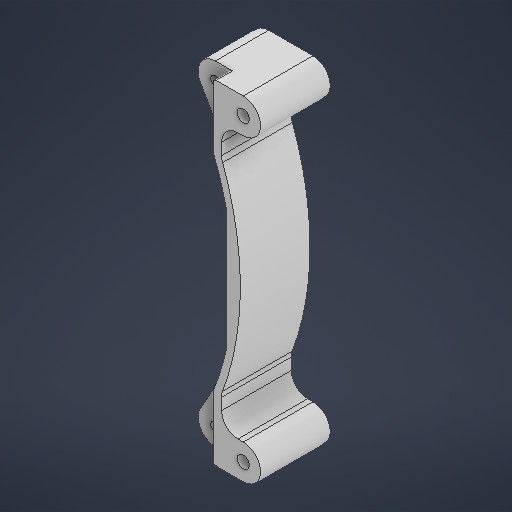
# Autodesk Inventor part: fan_connector_02
Saved by Autodesk Inventor 2026.2 (Build 302298010, 298A)
## iProperties
Created: 2026-05-14
Part Number: fan_connector_02
Material: 一般
Document SubType Name: Modeling
Designer: nyxeon
Density: 1 g/cm^3
Appearance: 既定
Author: nyxeon
Autodesk Inventor part; units mm, degrees
ref_plane "YZ Plane" through (0, 0, 0) normal (1, 0, 0) x (0, 1, 0)
ref_plane "XZ Plane" through (0, 0, 0) normal (0, 1, 0) x (-1, 0, 0)
ref_plane "XY Plane" through (0, 0, 0) normal (0, 0, 1) x (1, 0, 0)
sketch "スケッチ1" plane through (0, 0, 0) normal (0, 0, 1) x (1, 0, 0)
  line L0 (215.8192, 50.162) -> (210.8692, 50.162) construction
  line L1 (210.8692, 59.3371) -> (210.8692, 50.162) construction
  arc A0 (210.8692, 59.3371) -> (210.3611, 60.6691) centre (208.8692, 59.3371) ccw construction
  line L2 (208.3692, 62.9) -> (210.3611, 60.6691) construction
  line L3 (208.3692, 63.9) -> (208.3692, 62.9) construction
  arc A1 (206.8692, 65.4) -> (208.3692, 63.9) centre (208.3692, 65.4) ccw construction
  line L4 (206.8692, 65.4) -> (206.8692, 85.3) construction
  arc A2 (206.8692, 85.3) -> (200.8692, 91.3) centre (200.8692, 85.3) ccw construction
  line L5 (200.8692, 91.3) -> (180.9692, 91.3) construction
  arc A3 (179.4692, 92.8) -> (180.9692, 91.3) centre (180.9692, 92.8) ccw construction
  line L6 (179.4692, 92.8) -> (178.4692, 92.8) construction
  line L7 (178.4692, 92.8) -> (176.2383, 94.7919) construction
  arc A4 (176.2383, 94.7919) -> (174.9063, 95.3) centre (174.9063, 93.3) ccw construction
  line L8 (174.9063, 95.3) -> (153.3073, 95.3) construction
  arc A5 (153.3073, 95.3) -> (136.9278, 100.25) centre (115.5692, 0) ccw construction
  line L9 (94.2107, 100.25) -> (136.9278, 100.25) construction
  arc A6 (94.2107, 100.25) -> (77.8312, 95.3) centre (115.5692, 0) ccw construction
  line L10 (56.2322, 95.3) -> (77.8312, 95.3) construction
  arc A7 (56.2322, 95.3) -> (54.9001, 94.7919) centre (56.2322, 93.3) ccw construction
  line L11 (52.6692, 92.8) -> (54.9001, 94.7919) construction
  line L12 (51.6692, 92.8) -> (52.6692, 92.8) construction
  arc A8 (50.1692, 91.3) -> (51.6692, 92.8) centre (50.1692, 92.8) ccw construction
  line L13 (30.2692, 91.3) -> (50.1692, 91.3) construction
  arc A9 (30.2692, 91.3) -> (24.2692, 85.3) centre (30.2692, 85.3) ccw construction
  line L14 (24.2692, 65.4) -> (24.2692, 85.3) construction
  arc A10 (22.7692, 63.9) -> (24.2692, 65.4) centre (22.7692, 65.4) ccw construction
  line L15 (22.7692, 63.9) -> (22.7692, 62.9) construction
  line L16 (22.7692, 62.9) -> (20.7774, 60.6691) construction
  arc A11 (20.7774, 60.6691) -> (20.2692, 59.3371) centre (22.2692, 59.3371) ccw construction
  line L17 (20.2692, 59.3371) -> (20.2692, 37.738) construction
  arc A12 (20.2692, 37.738) -> (15.3192, 21.3585) centre (115.5692, 0) ccw construction
  line L18 (15.3192, -21.3585) -> (15.3192, 21.3585) construction
  arc A13 (15.3192, -21.3585) -> (20.2692, -37.738) centre (115.5692, 0) ccw construction
  line L19 (20.2692, -59.3371) -> (20.2692, -37.738) construction
  arc A14 (20.2692, -59.3371) -> (20.7774, -60.6691) centre (22.2692, -59.3371) ccw construction
  line L20 (22.7692, -62.9) -> (20.7774, -60.6691) construction
  line L21 (22.7692, -63.9) -> (22.7692, -62.9) construction
  arc A15 (24.2692, -65.4) -> (22.7692, -63.9) centre (22.7692, -65.4) ccw construction
  line L22 (24.2692, -65.4) -> (24.2692, -85.3) construction
  arc A16 (24.2692, -85.3) -> (30.2692, -91.3) centre (30.2692, -85.3) ccw construction
  line L23 (30.2692, -91.3) -> (50.1692, -91.3) construction
  arc A17 (51.6692, -92.8) -> (50.1692, -91.3) centre (50.1692, -92.8) ccw construction
  line L24 (51.6692, -92.8) -> (52.6692, -92.8) construction
  line L25 (52.6692, -92.8) -> (54.9001, -94.7919) construction
  arc A18 (54.9001, -94.7919) -> (56.2322, -95.3) centre (56.2322, -93.3) ccw construction
  line L26 (56.2322, -95.3) -> (77.8312, -95.3) construction
  arc A19 (77.8312, -95.3) -> (94.2107, -100.25) centre (115.5692, 0) ccw construction
  line L27 (94.2107, -100.25) -> (136.9278, -100.25) construction
  arc A20 (136.9278, -100.25) -> (153.3073, -95.3) centre (115.5692, 0) ccw construction
  line L28 (174.9063, -95.3) -> (153.3073, -95.3) construction
  arc A21 (174.9063, -95.3) -> (176.2383, -94.7919) centre (174.9063, -93.3) ccw construction
  line L29 (178.4692, -92.8) -> (176.2383, -94.7919) construction
  line L30 (179.4692, -92.8) -> (178.4692, -92.8) construction
  arc A22 (180.9692, -91.3) -> (179.4692, -92.8) centre (180.9692, -92.8) ccw construction
  line L31 (200.8692, -91.3) -> (180.9692, -91.3) construction
  arc A23 (200.8692, -91.3) -> (206.8692, -85.3) centre (200.8692, -85.3) ccw construction
  line L32 (206.8692, -65.4) -> (206.8692, -85.3) construction
  arc A24 (208.3692, -63.9) -> (206.8692, -65.4) centre (208.3692, -65.4) ccw construction
  line L33 (208.3692, -63.9) -> (208.3692, -62.9) construction
  line L34 (208.3692, -62.9) -> (210.3611, -60.6691) construction
  arc A25 (210.3611, -60.6691) -> (210.8692, -59.3371) centre (208.8692, -59.3371) ccw construction
  line L35 (210.8692, -59.3371) -> (210.8692, -37.738) construction
  arc A26 (210.8692, -37.738) -> (215.8192, -21.3585) centre (115.5692, 0) ccw construction
  line L36 (215.8192, -21.3585) -> (215.8192, 50.162) construction
  circle A27 centre (30.5692, 85) radius 2.2 construction
  circle A28 centre (38.3192, 77.25) radius 2.2 construction
  circle A29 centre (192.8192, -77.25) radius 2.2 construction
  circle A30 centre (200.5692, -85) radius 2.2 construction
  circle A31 centre (170.5692, -90) radius 2.2 construction
  circle A32 centre (200.5817, -67.0124) radius 1.35 construction
  circle A33 centre (205.5692, -55) radius 2.2 construction
  circle A34 centre (182.5817, 85.0124) radius 1.35 construction
  circle A35 centre (192.8192, 77.25) radius 2.2 construction
  circle A36 centre (200.5692, 85) radius 2.2 construction
  circle A37 centre (170.5692, 90) radius 2.2 construction
  circle A38 centre (200.5817, 67.0124) radius 1.35 construction
  circle A39 centre (205.5692, 55) radius 2.2 construction
  circle A40 centre (182.5817, -85.0124) radius 1.35 construction
  circle A41 centre (25.5692, -55) radius 2.2 construction
  circle A42 centre (30.5568, -67.0124) radius 1.35 construction
  circle A43 centre (60.5692, -90) radius 2.2 construction
  circle A44 centre (30.5692, -85) radius 2.2 construction
  circle A45 centre (60.5692, 90) radius 2.2 construction
  circle A46 centre (30.5568, 67.0124) radius 1.35 construction
  circle A47 centre (25.5692, 55) radius 2.2 construction
  circle A48 centre (48.5568, -85.0124) radius 1.35 construction
  circle A49 centre (48.5568, 85.0124) radius 1.35 construction
  circle A50 centre (38.3192, -77.25) radius 2.2 construction
  arc A51 (49.757, -72.8834) -> (93.3332, -95.6494) centre (115.5692, 0) ccw construction
  line L37 (49.757, -72.8834) -> (41.388, -81.2523) construction
  arc A52 (40.2566, -80.121) -> (41.388, -81.2523) centre (40.8223, -80.6866) ccw construction
  line L38 (48.5772, -71.8004) -> (40.2566, -80.121) construction
  arc A53 (43.7688, -66.9921) -> (48.5772, -71.8004) centre (115.5692, 0) ccw construction
  line L39 (43.7688, -66.9921) -> (35.4483, -75.3126) construction
  arc A54 (34.3169, -74.1813) -> (35.4483, -75.3126) centre (34.8826, -74.747) ccw construction
  line L40 (42.6859, -65.8123) -> (34.3169, -74.1813) construction
  arc A55 (19.9199, -22.236) -> (42.6859, -65.8123) centre (115.5692, 0) ccw construction
  line L41 (18.6687, -21) -> (19.9199, -22.236) construction
  arc A56 (18.6687, 21) -> (18.6687, -21) centre (115.5692, 0) ccw construction
  line L42 (18.6687, 21) -> (19.9199, 22.236) construction
  arc A57 (42.6859, 65.8123) -> (19.9199, 22.236) centre (115.5692, 0) ccw construction
  line L43 (42.6859, 65.8123) -> (34.3169, 74.1813) construction
  arc A58 (35.4483, 75.3126) -> (34.3169, 74.1813) centre (34.8826, 74.747) ccw construction
  line L44 (43.7688, 66.9921) -> (35.4483, 75.3126) construction
  arc A59 (48.5772, 71.8004) -> (43.7688, 66.9921) centre (115.5692, 0) ccw construction
  line L45 (48.5772, 71.8004) -> (40.2566, 80.121) construction
  arc A60 (41.388, 81.2523) -> (40.2566, 80.121) centre (40.8223, 80.6866) ccw construction
  line L46 (49.757, 72.8834) -> (41.388, 81.2523) construction
  arc A61 (93.3332, 95.6494) -> (49.757, 72.8834) centre (115.5692, 0) ccw construction
  line L47 (94.5692, 96.9006) -> (93.3332, 95.6494) construction
  arc A62 (136.5692, 96.9006) -> (94.5692, 96.9006) centre (115.5692, 0) ccw construction
  line L48 (136.5692, 96.9006) -> (137.8053, 95.6494) construction
  arc A63 (181.3815, 72.8834) -> (137.8053, 95.6494) centre (115.5692, 0) ccw construction
  line L49 (181.3815, 72.8834) -> (189.7505, 81.2523) construction
  arc A64 (190.8819, 80.121) -> (189.7505, 81.2523) centre (190.3162, 80.6866) ccw construction
  line L50 (182.5613, 71.8004) -> (190.8819, 80.121) construction
  arc A65 (187.3697, 66.9921) -> (182.5613, 71.8004) centre (115.5692, 0) ccw construction
  line L51 (187.3697, 66.9921) -> (195.6902, 75.3126) construction
  arc A66 (196.8216, 74.1813) -> (195.6902, 75.3126) centre (196.2559, 74.747) ccw construction
  line L52 (188.4526, 65.8123) -> (196.8216, 74.1813) construction
  arc A67 (211.2186, 22.236) -> (188.4526, 65.8123) centre (115.5692, 0) ccw construction
  line L53 (212.4698, 21) -> (211.2186, 22.236) construction
  arc A68 (212.4698, -21) -> (212.4698, 21) centre (115.5692, 0) ccw construction
  line L54 (212.4698, -21) -> (211.2186, -22.236) construction
  arc A69 (188.4526, -65.8123) -> (211.2186, -22.236) centre (115.5692, 0) ccw construction
  line L55 (188.4526, -65.8123) -> (196.8216, -74.1813) construction
  arc A70 (195.6902, -75.3126) -> (196.8216, -74.1813) centre (196.2559, -74.747) ccw construction
  line L56 (187.3697, -66.9921) -> (195.6902, -75.3126) construction
  arc A71 (182.5613, -71.8004) -> (187.3697, -66.9921) centre (115.5692, 0) ccw construction
  line L57 (182.5613, -71.8004) -> (190.8819, -80.121) construction
  arc A72 (189.7505, -81.2523) -> (190.8819, -80.121) centre (190.3162, -80.6866) ccw construction
  line L58 (181.3815, -72.8834) -> (189.7505, -81.2523) construction
  arc A73 (137.8053, -95.6494) -> (181.3815, -72.8834) centre (115.5692, 0) ccw construction
  line L59 (136.5692, -96.9006) -> (137.8053, -95.6494) construction
  arc A74 (94.5692, -96.9006) -> (136.5692, -96.9006) centre (115.5692, 0) ccw construction
  line L60 (94.5692, -96.9006) -> (93.3332, -95.6494) construction
  line L61 (12.0692, 50.162) -> (7.1192, 50.162) construction
  line L62 (7.1192, 59.3371) -> (7.1192, 50.162) construction
  arc A75 (7.1192, 59.3371) -> (6.6111, 60.6691) centre (5.1192, 59.3371) ccw construction
  line L63 (4.6192, 62.9) -> (6.6111, 60.6691) construction
  line L64 (4.6192, 63.9) -> (4.6192, 62.9) construction
  arc A76 (3.1192, 65.4) -> (4.6192, 63.9) centre (4.6192, 65.4) ccw construction
  line L65 (3.1192, 65.4) -> (3.1192, 85.3) construction
  arc A77 (3.1192, 85.3) -> (-2.8808, 91.3) centre (-2.8808, 85.3) ccw construction
  line L66 (-2.8808, 91.3) -> (-22.7808, 91.3) construction
  arc A78 (-24.2808, 92.8) -> (-22.7808, 91.3) centre (-22.7808, 92.8) ccw construction
  line L67 (-24.2808, 92.8) -> (-25.2808, 92.8) construction
  line L68 (-25.2808, 92.8) -> (-27.5117, 94.7919) construction
  arc A79 (-27.5117, 94.7919) -> (-28.8437, 95.3) centre (-28.8437, 93.3) ccw construction
  line L69 (-28.8437, 95.3) -> (-50.4427, 95.3) construction
  arc A80 (-50.4427, 95.3) -> (-66.8222, 100.25) centre (-88.1808, 0) ccw construction
  line L70 (-109.5393, 100.25) -> (-66.8222, 100.25) construction
  arc A81 (-109.5393, 100.25) -> (-125.9188, 95.3) centre (-88.1808, 0) ccw construction
  line L71 (-147.5178, 95.3) -> (-125.9188, 95.3) construction
  arc A82 (-147.5178, 95.3) -> (-148.8499, 94.7919) centre (-147.5178, 93.3) ccw construction
  line L72 (-151.0808, 92.8) -> (-148.8499, 94.7919) construction
  line L73 (-152.0808, 92.8) -> (-151.0808, 92.8) construction
  arc A83 (-153.5808, 91.3) -> (-152.0808, 92.8) centre (-153.5808, 92.8) ccw construction
  line L74 (-173.4808, 91.3) -> (-153.5808, 91.3) construction
  arc A84 (-173.4808, 91.3) -> (-179.4808, 85.3) centre (-173.4808, 85.3) ccw construction
  line L75 (-179.4808, 65.4) -> (-179.4808, 85.3) construction
  arc A85 (-180.9808, 63.9) -> (-179.4808, 65.4) centre (-180.9808, 65.4) ccw construction
  line L76 (-180.9808, 63.9) -> (-180.9808, 62.9) construction
  line L77 (-180.9808, 62.9) -> (-182.9726, 60.6691) construction
  arc A86 (-182.9726, 60.6691) -> (-183.4808, 59.3371) centre (-181.4808, 59.3371) ccw construction
  line L78 (-183.4808, 59.3371) -> (-183.4808, 37.738) construction
  arc A87 (-183.4808, 37.738) -> (-188.4308, 21.3585) centre (-88.1808, 0) ccw construction
  line L79 (-188.4308, -21.3585) -> (-188.4308, 21.3585) construction
  arc A88 (-188.4308, -21.3585) -> (-183.4808, -37.738) centre (-88.1808, 0) ccw construction
  line L80 (-183.4808, -59.3371) -> (-183.4808, -37.738) construction
  arc A89 (-183.4808, -59.3371) -> (-182.9726, -60.6691) centre (-181.4808, -59.3371) ccw construction
  line L81 (-180.9808, -62.9) -> (-182.9726, -60.6691) construction
  line L82 (-180.9808, -63.9) -> (-180.9808, -62.9) construction
  arc A90 (-179.4808, -65.4) -> (-180.9808, -63.9) centre (-180.9808, -65.4) ccw construction
  line L83 (-179.4808, -65.4) -> (-179.4808, -85.3) construction
  arc A91 (-179.4808, -85.3) -> (-173.4808, -91.3) centre (-173.4808, -85.3) ccw construction
  line L84 (-173.4808, -91.3) -> (-153.5808, -91.3) construction
  arc A92 (-152.0808, -92.8) -> (-153.5808, -91.3) centre (-153.5808, -92.8) ccw construction
  line L85 (-152.0808, -92.8) -> (-151.0808, -92.8) construction
  line L86 (-151.0808, -92.8) -> (-148.8499, -94.7919) construction
  arc A93 (-148.8499, -94.7919) -> (-147.5178, -95.3) centre (-147.5178, -93.3) ccw construction
  line L87 (-147.5178, -95.3) -> (-125.9188, -95.3) construction
  arc A94 (-125.9188, -95.3) -> (-109.5393, -100.25) centre (-88.1808, 0) ccw construction
  line L88 (-109.5393, -100.25) -> (-66.8222, -100.25) construction
  arc A95 (-66.8222, -100.25) -> (-50.4427, -95.3) centre (-88.1808, 0) ccw construction
  line L89 (-28.8437, -95.3) -> (-50.4427, -95.3) construction
  arc A96 (-28.8437, -95.3) -> (-27.5117, -94.7919) centre (-28.8437, -93.3) ccw construction
  line L90 (-25.2808, -92.8) -> (-27.5117, -94.7919) construction
  line L91 (-24.2808, -92.8) -> (-25.2808, -92.8) construction
  arc A97 (-22.7808, -91.3) -> (-24.2808, -92.8) centre (-22.7808, -92.8) ccw construction
  line L92 (-2.8808, -91.3) -> (-22.7808, -91.3) construction
  arc A98 (-2.8808, -91.3) -> (3.1192, -85.3) centre (-2.8808, -85.3) ccw construction
  line L93 (3.1192, -65.4) -> (3.1192, -85.3) construction
  arc A99 (4.6192, -63.9) -> (3.1192, -65.4) centre (4.6192, -65.4) ccw construction
  line L94 (4.6192, -63.9) -> (4.6192, -62.9) construction
  line L95 (4.6192, -62.9) -> (6.6111, -60.6691) construction
  arc A100 (6.6111, -60.6691) -> (7.1192, -59.3371) centre (5.1192, -59.3371) ccw construction
  line L96 (7.1192, -59.3371) -> (7.1192, -37.738) construction
  arc A101 (7.1192, -37.738) -> (12.0692, -21.3585) centre (-88.1808, 0) ccw construction
  line L97 (12.0692, -21.3585) -> (12.0692, 50.162) construction
  circle A102 centre (-173.1808, 85) radius 2.2 construction
  circle A103 centre (-165.4308, 77.25) radius 2.2 construction
  circle A104 centre (-10.9308, -77.25) radius 2.2 construction
  circle A105 centre (-3.1808, -85) radius 2.2 construction
  circle A106 centre (-33.1808, -90) radius 2.2 construction
  circle A107 centre (-3.1683, -67.0124) radius 1.35 construction
  circle A108 centre (1.8192, -55) radius 2.2 construction
  circle A109 centre (-21.1683, 85.0124) radius 1.35 construction
  circle A110 centre (-10.9308, 77.25) radius 2.2 construction
  circle A111 centre (-3.1808, 85) radius 2.2 construction
  circle A112 centre (-33.1808, 90) radius 2.2 construction
  circle A113 centre (-3.1683, 67.0124) radius 1.35 construction
  circle A114 centre (1.8192, 55) radius 2.2 construction
  circle A115 centre (-21.1683, -85.0124) radius 1.35 construction
  circle A116 centre (-178.1808, -55) radius 2.2 construction
  circle A117 centre (-173.1932, -67.0124) radius 1.35 construction
  circle A118 centre (-143.1808, -90) radius 2.2 construction
  circle A119 centre (-173.1808, -85) radius 2.2 construction
  circle A120 centre (-143.1808, 90) radius 2.2 construction
  circle A121 centre (-173.1932, 67.0124) radius 1.35 construction
  circle A122 centre (-178.1808, 55) radius 2.2 construction
  circle A123 centre (-155.1932, -85.0124) radius 1.35 construction
  circle A124 centre (-155.1932, 85.0124) radius 1.35 construction
  circle A125 centre (-165.4308, -77.25) radius 2.2 construction
  arc A126 (-153.993, -72.8834) -> (-110.4168, -95.6494) centre (-88.1808, 0) ccw construction
  line L98 (-153.993, -72.8834) -> (-162.362, -81.2523) construction
  arc A127 (-163.4934, -80.121) -> (-162.362, -81.2523) centre (-162.9277, -80.6866) ccw construction
  line L99 (-155.1728, -71.8004) -> (-163.4934, -80.121) construction
  arc A128 (-159.9812, -66.9921) -> (-155.1728, -71.8004) centre (-88.1808, 0) ccw construction
  line L100 (-159.9812, -66.9921) -> (-168.3017, -75.3126) construction
  arc A129 (-169.4331, -74.1813) -> (-168.3017, -75.3126) centre (-168.8674, -74.747) ccw construction
  line L101 (-161.0641, -65.8123) -> (-169.4331, -74.1813) construction
  arc A130 (-183.8301, -22.236) -> (-161.0641, -65.8123) centre (-88.1808, 0) ccw construction
  line L102 (-185.0813, -21) -> (-183.8301, -22.236) construction
  arc A131 (-185.0813, 21) -> (-185.0813, -21) centre (-88.1808, 0) ccw construction
  line L103 (-185.0813, 21) -> (-183.8301, 22.236) construction
  arc A132 (-161.0641, 65.8123) -> (-183.8301, 22.236) centre (-88.1808, 0) ccw construction
  line L104 (-161.0641, 65.8123) -> (-169.4331, 74.1813) construction
  arc A133 (-168.3017, 75.3126) -> (-169.4331, 74.1813) centre (-168.8674, 74.747) ccw construction
  line L105 (-159.9812, 66.9921) -> (-168.3017, 75.3126) construction
  arc A134 (-155.1728, 71.8004) -> (-159.9812, 66.9921) centre (-88.1808, 0) ccw construction
  line L106 (-155.1728, 71.8004) -> (-163.4934, 80.121) construction
  arc A135 (-162.362, 81.2523) -> (-163.4934, 80.121) centre (-162.9277, 80.6866) ccw construction
  line L107 (-153.993, 72.8834) -> (-162.362, 81.2523) construction
  arc A136 (-110.4168, 95.6494) -> (-153.993, 72.8834) centre (-88.1808, 0) ccw construction
  line L108 (-109.1808, 96.9006) -> (-110.4168, 95.6494) construction
  arc A137 (-67.1808, 96.9006) -> (-109.1808, 96.9006) centre (-88.1808, 0) ccw construction
  line L109 (-67.1808, 96.9006) -> (-65.9447, 95.6494) construction
  arc A138 (-22.3685, 72.8834) -> (-65.9447, 95.6494) centre (-88.1808, 0) ccw construction
  line L110 (-22.3685, 72.8834) -> (-13.9995, 81.2523) construction
  arc A139 (-12.8681, 80.121) -> (-13.9995, 81.2523) centre (-13.4338, 80.6866) ccw construction
  line L111 (-21.1887, 71.8004) -> (-12.8681, 80.121) construction
  arc A140 (-16.3803, 66.9921) -> (-21.1887, 71.8004) centre (-88.1808, 0) ccw construction
  line L112 (-16.3803, 66.9921) -> (-8.0598, 75.3126) construction
  arc A141 (-6.9284, 74.1813) -> (-8.0598, 75.3126) centre (-7.4941, 74.747) ccw construction
  line L113 (-15.2974, 65.8123) -> (-6.9284, 74.1813) construction
  arc A142 (7.4686, 22.236) -> (-15.2974, 65.8123) centre (-88.1808, 0) ccw construction
  line L114 (8.7198, 21) -> (7.4686, 22.236) construction
  arc A143 (8.7198, -21) -> (8.7198, 21) centre (-88.1808, 0) ccw construction
  line L115 (8.7198, -21) -> (7.4686, -22.236) construction
  arc A144 (-15.2974, -65.8123) -> (7.4686, -22.236) centre (-88.1808, 0) ccw construction
  line L116 (-15.2974, -65.8123) -> (-6.9284, -74.1813) construction
  arc A145 (-8.0598, -75.3126) -> (-6.9284, -74.1813) centre (-7.4941, -74.747) ccw construction
  line L117 (-16.3803, -66.9921) -> (-8.0598, -75.3126) construction
  arc A146 (-21.1887, -71.8004) -> (-16.3803, -66.9921) centre (-88.1808, 0) ccw construction
  line L118 (-21.1887, -71.8004) -> (-12.8681, -80.121) construction
  arc A147 (-13.9995, -81.2523) -> (-12.8681, -80.121) centre (-13.4338, -80.6866) ccw construction
  line L119 (-22.3685, -72.8834) -> (-13.9995, -81.2523) construction
  arc A148 (-65.9447, -95.6494) -> (-22.3685, -72.8834) centre (-88.1808, 0) ccw construction
  line L120 (-67.1808, -96.9006) -> (-65.9447, -95.6494) construction
  arc A149 (-109.1808, -96.9006) -> (-67.1808, -96.9006) centre (-88.1808, 0) ccw construction
  line L121 (-109.1808, -96.9006) -> (-110.4168, -95.6494) construction
  arc A150 (-14.8018, -66.3079) -> (8.3934, -21.3225) centre (-88.1808, 0) ccw construction
  arc A151 (18.9951, -21.3225) -> (42.1903, -66.3079) centre (115.5692, 0) ccw construction
  line L122 (-88.1808, 0) -> (115.5692, 0) construction
  circle A152 centre (1.8192, -55) radius 6.3251 construction
  circle A153 centre (25.5692, -55) radius 6.3251 construction
  arc A154 (18.6687, -21) -> (94.5692, -96.9006) centre (115.5692, 0) ccw construction
  circle A155 centre (1.8192, 55) radius 6.3251 construction
  circle A156 centre (25.5692, 55) radius 6.3251 construction
  line L123 (25.5692, -55) -> (115.5692, 0) construction
  arc A157 (30.9663, 51.7018) -> (30.9663, -51.7018) centre (115.5692, 0) ccw
  arc A158 (-3.5779, -51.7018) -> (-3.5779, 51.7018) centre (-88.1808, 0) ccw
  arc A159 (25.5692, -61.3251) -> (30.9663, -51.7018) centre (25.5692, -55) ccw
  arc A160 (-3.5779, -51.7018) -> (1.8192, -61.3251) centre (1.8192, -55) ccw
  arc A161 (1.8192, 61.3251) -> (-3.5779, 51.7018) centre (1.8192, 55) ccw
  arc A162 (30.9663, 51.7018) -> (25.5692, 61.3251) centre (25.5692, 55) ccw
  line L124 (1.8192, -61.3251) -> (25.5692, -61.3251)
  line L125 (1.8192, 61.3251) -> (25.5692, 61.3251)
  circle A163 centre (1.8192, -55) radius 1.7
  circle A164 centre (25.5692, -55) radius 1.7
  circle A165 centre (25.5692, 55) radius 1.7
  circle A166 centre (1.8192, 55) radius 1.7
  line L126 (16.4192, 61.3251) -> (16.4192, -61.3251)
  point P0 (0, 0)
  dimension "d0" = 12.6502
  dimension "d1" = 3.4
  constraints: 26 point on circle, 16 centre point, 15 coincident, 10 end point, 5 equal radius, 3 concentric, 3 point on line, 3 tangent, 2 horizontal, 1 horizontal alignment, 1 parallel, 1 vertical, 1 vertical alignment, 11 other
  measures "d0" diameter of A152
  measures "d1" diameter of A163
extrude "押し出し1" add sketch "スケッチ1" along normal blind 15.8 and the other way blind 3.8 contours L126 L124 A160 A158 A161 L125
sketch "スケッチ2" plane through (0, 0, 15.8) normal (0, 0, 1) x (1, 0, 0)
  arc A0 (-270.5722, -100.25) -> (-254.1927, -95.3) centre (-291.9308, 0) ccw construction
  circle A1 centre (18.0692, -55) radius 2.25
  line L0 (7.1192, -59.3371) -> (7.1192, -37.738) projected
  arc A2 (7.1192, -37.738) -> (12.0692, -21.3585) centre (-88.1808, 0) ccw projected
  line L1 (12.0692, -21.3585) -> (12.0692, 21.3585) projected
  arc A3 (12.0692, 21.3585) -> (7.1192, 37.738) centre (-88.1808, 0) ccw projected
  line L2 (7.1192, 59.3371) -> (7.1192, 37.738) projected
  arc A4 (7.1192, 59.3371) -> (6.6111, 60.6691) centre (5.1192, 59.3371) ccw projected
  line L3 (4.6192, 62.9) -> (6.6111, 60.6691) projected
  arc A5 (6.6111, -60.6691) -> (7.1192, -59.3371) centre (5.1192, -59.3371) ccw projected
  line L4 (4.6192, -62.9) -> (6.6111, -60.6691) projected
  line L5 (16.4192, -61.3251) -> (16.4192, 61.3251) projected
  line L6 (16.4192, 61.3251) -> (1.8192, 61.3251) projected
  line L7 (1.8192, -61.3251) -> (16.4192, -61.3251) projected
  circle A6 centre (1.8192, -55) radius 1.7 construction
  circle A7 centre (1.8192, 55) radius 1.7 construction
  arc A8 (-3.5779, -51.7018) -> (1.8192, -61.3251) centre (1.8192, -55) ccw construction
  circle A9 centre (18.0692, -55) radius 6.3251 construction
  line L8 (16.4192, -61.3251) -> (18.0692, -61.3251)
  line L9 (7.1192, -59.3371) -> (7.1192, -61.3251)
  circle A10 centre (18.0692, 55) radius 2.25
  circle A11 centre (18.0692, 55) radius 6.3251 construction
  line L10 (7.1192, 59.3371) -> (7.1192, 61.3251)
  line L11 (16.4192, 61.3251) -> (18.0692, 61.3251)
  line L12 (24.3944, 55) -> (24.3944, -55)
  arc A12 (24.3944, 55) -> (18.0692, 61.3251) centre (18.0692, 55) ccw
  arc A13 (18.0692, -61.3251) -> (24.3944, -55) centre (18.0692, -55) ccw
  point P0 (0, 0)
  dimension "d8" = 310
  dimension "d9" = 4.5
  constraints: 10 end point, 8 point on circle, 6 centre point, 4 coincident, 4 tangent, 3 equal radius, 2 horizontal alignment, 2 point on line, 1 perpendicular, 1 vertical, 1 vertical alignment
  measures "d8" horizontal distance of A1.centre A0.centre
  measures "d9" diameter of A1
extrude "押し出し2" add sketch "スケッチ2" along normal blind 6 contours A1 L5 A10 L11 A12 L12 A13 L8 | A1 L5 L7 L9 L0 A2 L1 A3 L2 L10 L6 A10
sketch "スケッチ3" plane through (0, 0, -3.8) normal (0, 0, -1) x (-1, 0, 0)
  circle A0 centre (-18.0692, 55) radius 2.25 projected
  circle A1 centre (-18.0692, -55) radius 2.25 projected
  point P0 (0, 0)
extrude "押し出し3" cut sketch "スケッチ3" against normal through all
sketch "スケッチ4" plane through (0, 0, 15.8) normal (0, 0, -1) x (-1, 0, 0)
  line L0 (-16.4192, 56.5297) -> (-16.4192, 61.3251) projected
  line L1 (-18.0692, 61.3251) -> (-16.4192, 61.3251) projected
  arc A0 (-18.0692, 61.3251) -> (-24.3944, 55) centre (-18.0692, 55) ccw projected
  line L2 (-24.3944, -55) -> (-24.3944, 55) projected
  arc A1 (-24.3944, -55) -> (-18.0692, -61.3251) centre (-18.0692, -55) ccw projected
  line L3 (-16.4192, -61.3251) -> (-18.0692, -61.3251) projected
  line L4 (-16.4192, -61.3251) -> (-16.4192, -56.5297) projected
  arc A2 (-16.4192, -53.4703) -> (-16.4192, -56.5297) centre (-18.0692, -55) ccw projected
  line L5 (-16.4192, -53.4703) -> (-16.4192, 53.4703) projected
  arc A3 (-16.4192, 56.5297) -> (-16.4192, 53.4703) centre (-18.0692, 55) ccw projected
  point P0 (0, 0)
extrude "押し出し4" add sketch "スケッチ4" along normal up to surface (19.6 mm away)
sketch "スケッチ5" plane through (0, 0, -3.8) normal (0, 0, -1) x (-1, 0, 0)
  circle A0 centre (-18.0692, -55) radius 2.25 construction
  circle A1 centre (-18.0692, 55) radius 2.25 construction
  circle A2 centre (-18.0692, -55) radius 4.1
  circle A3 centre (-18.0692, 55) radius 4.1
  point P0 (0, 0)
  dimension "d16" = 8.2
  constraints: 2 centre point, 2 coincident, 1 equal radius
  measures "d16" diameter of A2
extrude "押し出し5" cut sketch "スケッチ5" against normal blind 21.6
sketch "スケッチ6" plane through (0, 0, 21.8) normal (0, 0, 1) x (1, 0, 0)
  arc A0 (-3.5779, -51.7018) -> (1.8192, -61.3251) centre (1.8192, -55) ccw projected
  line L0 (1.8192, -61.3251) -> (7.1192, -61.3251) projected
  line L1 (7.1192, -61.3251) -> (18.0692, -61.3251) projected
  arc A1 (18.0692, -61.3251) -> (24.3944, -55) centre (18.0692, -55) ccw projected
  arc A2 (-3.5779, -51.7018) -> (-3.5779, 51.7018) centre (-88.1808, 0) ccw projected
  arc A3 (1.8192, 61.3251) -> (-3.5779, 51.7018) centre (1.8192, 55) ccw projected
  line L2 (7.1192, 61.3251) -> (1.8192, 61.3251) projected
  line L3 (18.0692, 61.3251) -> (7.1192, 61.3251) projected
  arc A4 (24.3944, 55) -> (18.0692, 61.3251) centre (18.0692, 55) ccw projected
  arc A5 (5.0248, -48.6749) -> (5.0248, 48.6749) centre (-88.1808, 0) ccw
  arc A6 (24.3944, -55) -> (18.0692, -48.6749) centre (18.0692, -55) ccw
  line L4 (18.0692, -48.6749) -> (5.0248, -48.6749)
  line L5 (10.1192, -48.6749) -> (10.1192, -37.3314)
  line L6 (7.1192, -37.738) -> (7.1192, -61.3251) construction
  circle A7 centre (18.0692, 55) radius 2.25 construction
  arc A8 (18.0692, 48.6749) -> (24.3944, 55) centre (18.0692, 55) ccw
  line L7 (18.0692, 48.6749) -> (5.0248, 48.6749)
  line L8 (10.1192, 48.6749) -> (10.1192, 37.3314)
  line L9 (7.1192, 61.3251) -> (7.1192, 37.738) construction
  point P0 (0, 0)
  dimension "d19" = 6
  dimension "d20" = 3
  dimension "d21" = 3
  constraints: 8 end point, 8 point on circle, 3 centre point, 3 coincident, 2 horizontal, 2 point on line, 2 tangent, 2 vertical
  measures "d19" radial gap between concentric circles of A2 A5
  measures "d20" distance between parallel lines of L6 L5
  measures "d21" distance between parallel lines of L9 L8
extrude "押し出し6" cut sketch "スケッチ6" against normal through all keep common part
fillet "フィレット2" radius 6 4 edges at (10.1192, 48.6749, 9) (10.1192, 37.3314, 9) (10.1192, -37.3314, 9) (10.1192, -48.6749, 9)
fillet "フィレット2" radius 1 4 edges at (7.1192, 61.3251, 18.8) (7.1192, 37.738, 18.8) (7.1192, -37.738, 18.8) (7.1192, -61.3251, 18.8)
